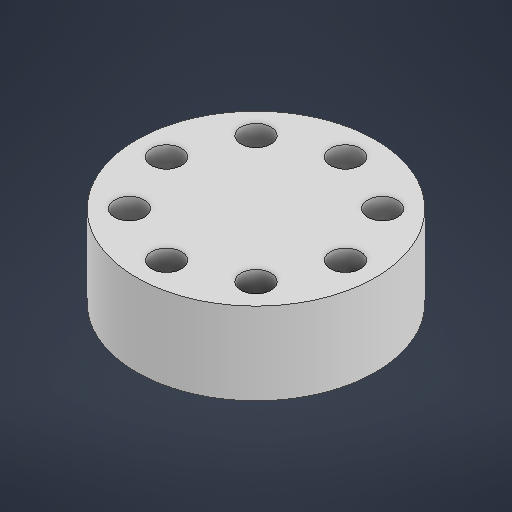
# Autodesk Inventor part: ArmBearingSpacer2
Saved by Autodesk Inventor 2025 (Build 290162000, 162)
## iProperties
Created: 2024-05-20
Part Number: ArmBearingSpacer2
Material: Generic
Document SubType Name: Modeling
Designer: avsar
Density: 1 g/cm^3
Appearance: Default
Author: avsar
Autodesk Inventor part; units mm, degrees
ref_plane "YZ Plane" through (0, 0, 0) normal (1, 0, 0) x (0, 1, 0)
ref_plane "XZ Plane" through (0, 0, 0) normal (0, 1, 0) x (-1, 0, 0)
ref_plane "XY Plane" through (0, 0, 0) normal (0, 0, 1) x (1, 0, 0)
sketch "Sketch1" plane through (0, 0, 0) normal (0, 1, 0) x (-1, 0, 0)
  circle A0 centre (0, 0) radius 16
  circle A1 centre (0, -12) radius 2
  circle A2 centre (8.4853, -8.4853) radius 2
  circle A3 centre (12, 0) radius 2
  circle A4 centre (8.4853, 8.4853) radius 2
  circle A5 centre (0, 12) radius 2
  circle A6 centre (-8.4853, 8.4853) radius 2
  circle A7 centre (-12, 0) radius 2
  circle A8 centre (-8.4853, -8.4853) radius 2
  dimension "d0" = 32
  dimension "d1" = 4
  dimension "d2" = 12
  dimension "d5" = 360
  constraints: 9 centre point, 1 coincident, 1 vertical alignment, 17 other
  measures "d0" diameter of A0
  measures "d1" diameter of A1
  measures "d2" distance of point (0, 0) A1.centre
extrude "Extrusion1" add sketch "Sketch1" along normal blind 11
body "Solid1"
